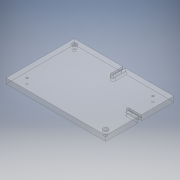
# Autodesk Inventor part: PCB FIxture 160x100
Saved by Autodesk Inventor 2017 (Build 210142000, 142)
## iProperties
Created: 2016-09-16
Part Number: PCB FIxture 160x100
Material: Polycarbonate, Clear
Document SubType Name: Modeling
Designer: Andreas Fröderberg
Density: 1.2 g/cm^3
Appearance: Polycarbonate - Clear
Author: Andreas Fröderberg
Autodesk Inventor part; units mm, degrees
ref_plane "YZ Plane" through (0, 0, 0) normal (1, 0, 0) x (0, 1, 0)
ref_plane "XZ Plane" through (0, 0, 0) normal (0, 1, 0) x (-1, 0, 0)
ref_plane "XY Plane" through (0, 0, 0) normal (0, 0, 1) x (1, 0, 0)
sketch "Sketch1" plane through (0, 0, 0) normal (0, 0, 1) x (1, 0, 0)
  line L0 (-20, -20) -> (170, -20)
  line L1 (170, -20) -> (170, 110)
  line L2 (170, 110) -> (-20, 110)
  line L3 (-20, 110) -> (-20, -20)
  point P0 (0, 0)
  dimension "W_tot" = 190
  dimension "H_tot" = 130
  dimension "E_to_Hole_X" = 20
  dimension "E_to_Hole_Y" = 20
  constraints: 8 end point, 2 parallel, 1 horizontal, 1 perpendicular
  measures "W_tot" distance of L1.end L2.end
  measures "H_tot" distance of L2.end L0.start
  measures "E_to_Hole_X" distance from line of L3 point (0, 0)
  measures "E_to_Hole_Y" distance from line of L0 point (0, 0)
extrude "Body_Ex" add sketch "Sketch1" against normal blind 10
sketch "Hole_4_sk" plane through (0, 0, 0) normal (0, 0, 1) x (1, 0, 0)
  line L0 (0, 0) -> (150, 0) construction
  line L1 (150, 0) -> (150, 90) construction
  line L2 (150, 90) -> (0, 90) construction
  line L3 (0, 90) -> (0, 0) construction
  dimension "CP_Hole_X" = 150
  dimension "CP_Hole_Y" = 90
  constraints: 8 end point, 2 coincident, 2 parallel, 1 horizontal, 1 perpendicular
  measures "CP_Hole_X" distance of L1.end L2.end
  measures "CP_Hole_Y" distance of L0.end L1.end
hole "Hole1" at (150, 90, 0) at (0, 0, 0) direction (0, 0, -1) diameter 4 end through all
sketch "Lock Track Profile" plane through (170, -20, 0) normal (1, 0, 0) x (0, 0, -1)
  line L0 (0, 62.4) -> (5, 62.4)
  line L1 (5, 62.4) -> (5, 60.9)
  line L2 (5, 60.9) -> (10, 60.9)
  line L3 (10, 60.9) -> (10, 69.1)
  line L4 (10, 69.1) -> (5, 69.1)
  line L5 (5, 69.1) -> (5, 67.6)
  line L6 (5, 67.6) -> (0, 67.6)
  line L7 (0, 67.6) -> (0, 62.4)
  line L8 (0, 0) -> (0, 130) projected
  line L9 (10, 130) -> (10, 0) projected
  point P0 (0, 20)
  dimension "Lock_Track_W" = 5.2
  dimension "Lock_Track_Bolt_W" = 8.2
  dimension "Origin_to_lock_track" = 40.9
  constraints: 16 end point, 6 perpendicular, 2 collinear, 2 equal length, 2 horizontal, 1 vertical alignment
  measures "Lock_Track_W" distance of L6.end L0.start
  measures "Lock_Track_Bolt_W" distance of L2.end L3.end
  measures "Origin_to_lock_track" distance from line of L2 point (0, 20)
sketch "Sketch5" plane through (0, 0, 0) normal (0, 0, 1) x (1, 0, 0)
  line L0 (145, 45) -> (170, 45)
  line L1 (170, -20) -> (170, 110) projected
  circle A0 centre (150, 90) radius 2 projected
  point P0 (0, 0)
  dimension "d19" = 45
  dimension "d20" = 5
  constraints: 2 end point, 1 horizontal, 1 midpoint
  measures "d19" distance from line of L0 point (0, 0)
  measures "d20" horizontal distance of L0.start A0.centre
sweep "Lock track" cut profiles "Lock Track Profile" path "Sketch5" path curves L0
full round fillet "Lock track fillet small" first side at (161.6667, 47.6, -3.3333) centre faces at (145, 45.8667, -8.3333) second side at (161.6667, 42.4, -1.6667)
full round fillet "Lock track fillet large" first side at (161.6667, 49.1, -8.3333) centre faces at (145, 45, -8.3333) second side at (161.6667, 40.9, -6.6667)
sketch "Lock track Y" plane through (-20, 110, 0) normal (0, 1, 0) x (1, 0, 0)
  line L0 (97.6, 0) -> (92.4, 0)
  line L1 (92.4, 0) -> (92.4, 5)
  line L2 (92.4, 5) -> (90.9, 5)
  line L3 (90.9, 5) -> (90.9, 10)
  line L4 (90.9, 10) -> (99.1, 10)
  line L5 (99.1, 10) -> (99.1, 5)
  line L6 (99.1, 5) -> (97.6, 5)
  line L7 (97.6, 5) -> (97.6, 0)
  line L8 (0, 10) -> (190, 10) projected
  line L9 (190, 0) -> (0, 0) projected
  point P0 (20, 0)
  dimension "d23" = 8.2
  dimension "d24" = 5.2
  dimension "d25" = 5
  dimension "d26" = 70.9
  constraints: 16 end point, 6 perpendicular, 3 collinear, 2 point on line, 1 horizontal, 1 horizontal alignment
  measures "d23" distance of L3.end L4.end
  measures "d24" distance of L0.start L0.end
  measures "d25" distance of L4.end L5.end
  measures "d26" distance from line of L3 point (20, 0)
sketch "Lock track 2 Profile" plane through (0, 0, 0) normal (0, 0, 1) x (1, 0, 0)
  line L0 (75, 110) -> (75, 85)
  line L1 (170, 110) -> (-20, 110) projected
  circle A0 centre (150, 90) radius 2 projected
  point P0 (0, 0)
  dimension "d27" = 5
  dimension "d28" = 75
  constraints: 2 end point, 1 midpoint, 1 vertical
  measures "d27" vertical distance of L0.end A0.centre
  measures "d28" distance from line of point (0, 0) L0
sweep "Sweep2" cut profiles "Lock track Y" path "Lock track 2 Profile" path curves L0
full round fillet "Fillet3" first side at (77.6, 93.3333, -1.6667) centre faces at (75.8667, 85, -8.3333) second side at (72.4, 93.3333, -3.3333)
full round fillet "Fillet4" first side at (79.1, 93.3333, -6.6667) centre faces at (75, 85, -8.3333) second side at (70.9, 93.3333, -8.3333)
sketch "Sketch9" plane through (0, 0, 0) normal (0, 0, 1) x (1, 0, 0)
  line L0 (-20, 110) -> (-20, -20) projected
  line L1 (-20, 110) -> (70.9, 110) projected
  line L2 (-20, -20) -> (170, -20) projected
  line L3 (170, -20) -> (170, 42.4) projected
  point P0 (0, 0)
  point P1 (-10, 100)
  point P2 (160, -10)
  dimension "d31" = 10
  dimension "d32" = 10
  dimension "d33" = 10
  dimension "d34" = 10
  measures "d31" distance from line of L0 point (-10, 100)
  measures "d32" distance from line of L1 point (-10, 100)
  measures "d33" distance from line of point (160, -10) L2
  measures "d34" distance from line of point (160, -10) L3
hole "Hole2" at (-10, 100, 0) at (160, -10, 0) direction (0, 0, -1) diameter 5.7 end through all counterbore diameter 9.75 counterbore depth 5
equation "\"Origin_to_lock_track\" = 0.5 * CP_Hole_Y - 0.5 * Lock_Track_Bolt_W"
equation "\"d19\" = 0.5 * CP_Hole_Y"
equation "\"d23\" = Lock_Track_Bolt_W"
equation "\"d24\" = Lock_Track_W"
equation "\"d25\" = 0.5 * T_Base_Ex"
equation "\"d26\" = 0.5 * CP_Hole_X - 0.5 * Lock_Track_Bolt_W"
equation "\"d28\" = 0.5 * CP_Hole_X"
equation "\"T_Base_Ex\" = 10"
